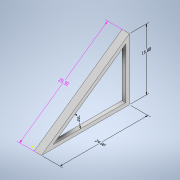
# Autodesk Inventor part: ballRampLeftSide-35degee-V04
Saved by Autodesk Inventor 2020.2 (Build 242310000, 310)
## iProperties
Created: 2020-01-24
Part Number: ballRampLeftSide-35degee-V04
Material: Generic
Document SubType Name: Modeling
Designer: robst
Density: 1 g/cm^3
Appearance: Default
Author: robst
Autodesk Inventor part; units mm, degrees
ref_plane "YZ Plane" through (0, 0, 0) normal (1, 0, 0) x (0, 1, 0)
ref_plane "XZ Plane" through (0, 0, 0) normal (0, 1, 0) x (-1, 0, 0)
ref_plane "XY Plane" through (0, 0, 0) normal (0, 0, 1) x (1, 0, 0)
sketch "Sketch1" plane through (0, 0, 0) normal (1, 0, 0) x (0, 1, 0)
  line L0 (0, 0) -> (0, -609.6)
  line L1 (0, -609.6) -> (426.8465, -609.6)
  line L2 (426.8465, -609.6) -> (0, 0)
  line L3 (25.4, -80.5585) -> (378.0536, -584.2)
  line L4 (378.0536, -584.2) -> (25.4, -584.2)
  line L5 (25.4, -584.2) -> (25.4, -80.5585)
  dimension "d0" = 609.6
  dimension "d1" = 35
  dimension "d2" = 25.4
  dimension "d3" = 25.4
  dimension "d4" = 25.4
  constraints: 12 end point, 2 parallel, 2 perpendicular, 1 horizontal, 1 vertical
  measures "d0" distance of L0.start L0.end
  measures "d1" angle of L2 L0
  measures "d2" distance between parallel lines of L3 L2
  measures "d3" distance between parallel lines of L5 L0
  measures "d4" distance between parallel lines of L4 L1
extrude "Extrusion1" add sketch "Sketch1" along normal mid plane 25.4
sketch "Sketch3" plane through (-12.7, 0, 0) normal (-1, 0, 0) x (0, 0, 1)
  line L0 (-609.6, 426.8465) -> (0, 0) projected
  line L1 (-609.6, 426.8465) -> (0, 0)
  line L2 (-80.5585, 25.4) -> (-584.2, 378.0536) projected
  line L3 (-584.2, 378.0536) -> (-44.2835, 0)
  line L4 (0, 0) -> (-609.6, 0) projected
  line L5 (-44.2835, 0) -> (0, 0)
  line L6 (0, 0) -> (-44.2835, 0)
  line L7 (-584.2, 378.0536) -> (-609.6, 395.8388)
  line L8 (-609.6, 0) -> (-609.6, 426.8465) projected
  line L9 (-609.6, 426.8465) -> (-609.6, 395.8388)
  constraints: 12 end point, 5 collinear, 2 point on line
extrude "Extrusion3" add sketch "Sketch3" along normal blind 25.4 contours L0 L4 L3 L2 L7 L8
ref_plane "powerCellWorkPlane" through (-38.1, 72.8226, 50.9909) normal (0, 0.819152, 0.5735764) x (1, 0, 0)
sketch "Sketch4" plane through (-38.1, 72.8226, 50.9909) normal (0, 0.819152, 0.5735764) x (1, 0, 0)
  point P0 (38.1, 0)
sketch "Sketch2" plane through (12.7, 0, 0) normal (1, 0, 0) x (0, 0, -1)
  line L0 (0, 0) -> (609.6, 0) projected
  line L1 (0, 0) -> (653.0822, 457.2931)
  line L2 (80.5585, 25.4) -> (584.2, 378.0536) projected
  line L3 (84.9829, 28.498) -> (584.2, 378.0536)
  line L4 (584.2, 378.0536) -> (662.4113, 432.8177)
  line L5 (584.2, 25.4) -> (80.5585, 25.4) projected
  line L6 (80.5585, 25.4) -> (44.2835, 0)
  line L7 (44.2835, 0) -> (0, 0)
  line L8 (609.6, 0) -> (609.6, 426.8465) projected
  line L9 (609.6, 426.8465) -> (609.6, 309.0206)
  point P0 (609.6, 511.5151)
  point P1 (68.5783, 24.3867)
  point P2 (69.7859, 25.4)
  constraints: 12 end point, 3 collinear, 2 point on line, 1 parallel, 1 other
body "Solid1"
